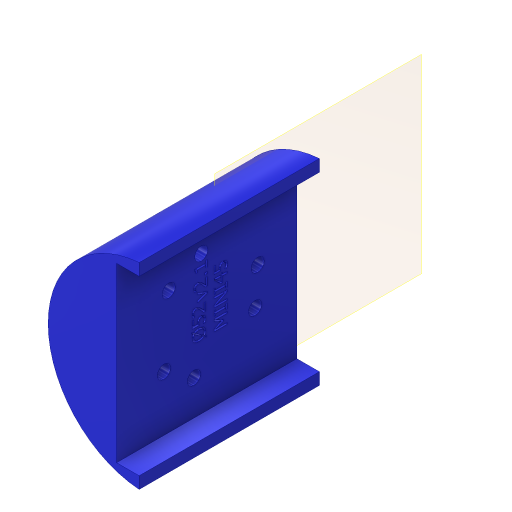
# Autodesk Inventor part: MINI45NewShell52v2-1_A
Saved by Autodesk Inventor 2023 (Build 270158000, 158)
## iProperties
Created: 2016-07-01
Part Number: MINI45NewShell52v2-1_A
Material: ABS Plastic
Document SubType Name: Modeling
Designer: Administrateur
Density: 1.06 g/cm^3
Appearance: Blue - Wall Paint - Glossy
Author: Administrateur
Autodesk Inventor part; units mm, degrees
ref_plane "XZ Plane" through (0, 0, 0) normal (0, 1, 0) x (-1, 0, 0)
sketch "Sketch1" plane through (0, 0, 0) normal (0, 0, 1) x (1, 0, 0)
  arc A0 (0, 26.2509) -> (0, -26.2509) centre (0, 0) ccw
  line L0 (0, 26.2509) -> (0, 23)
  line L1 (0, 23) -> (-8, 23)
  line L2 (-8, 23) -> (-8, 0)
  line L3 (-46.5484, 0) -> (26.4312, 0) construction
  line L4 (0, -26.2509) -> (0, -23)
  line L5 (0, -23) -> (-8, -23)
  line L6 (-8, -23) -> (-8, 0)
  dimension "d2" = 26.2509
  dimension "d3" = 46
  dimension "d4" = 8
  dimension "d27" = 23
  dimension "d28" = 3.2509
  constraints: 14 end point, 2 horizontal, 2 point on circle, 2 symmetric about line, 1 centre point, 1 coincident, 1 perpendicular, 1 vertical
  measures "d2" radius of A0
  measures "d3" distance between parallel lines of L5 L1
  measures "d4" distance of L0.end L1.end
  measures "d27" distance of L1.end L2.end
  measures "d28" distance of L0.start L0.end
extrude "Extrusion1" add sketch "Sketch1" along normal blind 120
sketch "Sketch2" plane through (-8, -23, 0) normal (1, 0, 0) x (0, 0, -1)
  line L0 (-60, 23) -> (-120, 23) construction
  line L1 (-120, 49.2509) -> (-120, -3.2509) construction
  line L2 (0, 49.2509) -> (-120, 49.2509) construction
  line L3 (-60, 49.2509) -> (-60, -3.2509) construction
  line L4 (0, -3.2509) -> (-120, -3.2509) construction
  line L5 (-60, 23) -> (-70.1427, 32.7947) construction
  circle A0 centre (-60, 23) radius 14.1 construction
  line L6 (-60, 23) -> (-61.4739, 37.0228) construction
  line L7 (-60, 23) -> (-63.4111, 9.3188) construction
  line L8 (-60, 23) -> (-71.4071, 14.7122) construction
  line L9 (-60, 23) -> (-46.4462, 26.8865) construction
  line L10 (-60, 23) -> (-47.119, 17.265) construction
  point P0 (0, 23)
  dimension "d32" = 28.2
  dimension "d34" = 40
  dimension "d37" = 360
  dimension "d39" = 84
  constraints: 16 end point, 11 coincident, 4 midpoint, 2 point on circle, 1 centre point, 17 other
  measures "d32" diameter of A0
  measures "d34" angle of L5 L6
  measures "d39" angle of L0 L6
hole "Hole1" at (-8, 14.0228, 61.4739) at (-8, 9.7947, 70.1427) at (-8, -8.2878, 71.4071) at (-8, -13.6812, 63.4111) at (-8, -5.735, 47.119) at (-8, 3.8865, 46.4462) direction (-1, 0, 0) diameter 3.5 end through all
ref_plane "Work Plane1" through (-26.2509, 0, 0) normal (1, 0, 0) x (0, 1, 0)
ref_plane "Work Plane2" through (-10, 0, 0) normal (1, 0, 0) x (0, 1, 0)
ref_plane "Work Plane3" through (-13.3, -23, 0) normal (1, 0, 0) x (0, 0, -1)
sketch "Sketch4" plane through (-13.3, -23, 0) normal (1, 0, 0) x (0, 0, -1)
  line L0 (0, 49.2509) -> (0, -3.2509) projected
  line L1 (0, -3.2509) -> (-120, -3.2509) projected
  line L2 (-120, 49.2509) -> (-120, -3.2509) projected
  line L3 (0, 49.2509) -> (-120, 49.2509) projected
  circle A0 centre (-61.4739, 37.0228) radius 1.75 projected
  circle A1 centre (-70.1427, 32.7947) radius 1.75 projected
  circle A2 centre (-71.4071, 14.7122) radius 1.75 projected
  circle A3 centre (-63.4111, 9.3188) radius 1.75 projected
  circle A4 centre (-47.119, 17.265) radius 1.75 projected
  circle A5 centre (-46.4462, 26.8865) radius 1.75 projected
  point P0 (0, 23)
  point P1 (-47.119, 19.015)
  point P2 (-71.4071, 16.4622)
  point P3 (-61.4739, 38.7728)
  point P4 (-70.1427, 34.5447)
  point P5 (-63.4111, 11.0688)
  point P6 (-46.4462, 28.6365)
  constraints: 6 coincident, 6 vertical alignment, 6 other
hole "Hole3" at (-13.3, 14.0228, 61.4739) at (-13.3, 9.7947, 70.1427) at (-13.3, -8.2878, 71.4071) at (-13.3, -13.6812, 63.4111) at (-13.3, -5.735, 47.119) at (-13.3, 3.8865, 46.4462) direction (-1, 0, 0) diameter 6.5 end through all
sketch "Sketch5" plane through (-8, -23, 0) normal (1, 0, 0) x (0, 0, -1)
  line L0 (-64.0358, 16.8519) -> (-64.0358, 25.5112) construction
  line L1 (-64.0358, 25.5112) -> (-65.8543, 25.5112) construction
  line L2 (-65.8543, 25.5112) -> (-65.8543, 16.8519) construction
  line L3 (-65.8543, 16.8519) -> (-64.0358, 16.8519) construction
  line L4 (-63.4273, 26.0588) -> (-63.4273, 31.0819) construction
  line L5 (-63.4273, 31.0819) -> (-59.8535, 31.0819) construction
  line L6 (-59.8535, 31.0819) -> (-59.8535, 26.0588) construction
  line L7 (-59.8535, 26.0588) -> (-63.4273, 26.0588) construction
  spline S0 degree 2 poles (-62.0703, 20.1023) (-61.2024, 20.1023) (-60.2465, 19.2571) (-60.2465, 18.5537) knots 0 0 0 1 2 2 2
  spline S1 degree 2 poles (-60.2465, 18.5537) (-60.2465, 18.2956) (-60.3827, 17.8503) (-60.5075, 17.6716) knots 0 0 0 1 2 2 2
  line L8 (-60.5075, 17.6716) -> (-60.048, 17.3596)
  line L9 (-60.048, 17.3596) -> (-60.048, 17.0136)
  line L10 (-60.048, 17.0136) -> (-60.7003, 17.4561)
  spline S2 degree 2 poles (-60.7003, 17.4561) (-60.9329, 17.2462) (-61.6193, 17.0079) (-62.0703, 17.0079) knots 0 0 0 1 2 2 2
  spline S3 degree 2 poles (-62.0703, 17.0079) (-62.9353, 17.0079) (-63.894, 17.856) (-63.894, 18.5537) knots 0 0 0 1 2 2 2
  spline S4 degree 2 poles (-63.894, 18.5537) (-63.894, 18.8231) (-63.7635, 19.2429) (-63.6359, 19.4301) knots 0 0 0 1 2 2 2
  line L11 (-63.6359, 19.4301) -> (-64.0358, 19.6996)
  line L12 (-64.0358, 19.6996) -> (-64.0358, 20.0484)
  line L13 (-64.0358, 20.0484) -> (-63.4459, 19.6457)
  spline S5 degree 2 poles (-63.4459, 19.6457) (-63.2133, 19.8612) (-62.5383, 20.1023) (-62.0703, 20.1023) knots 0 0 0 1 2 2 2
  spline S6 degree 2 poles (-62.0703, 19.623) (-62.3936, 19.623) (-62.9013, 19.4925) (-63.0686, 19.3847) knots 0 0 0 1 2 2 2
  line L14 (-63.0686, 19.3847) -> (-60.8648, 17.9099)
  spline S7 degree 2 poles (-60.8648, 17.9099) (-60.7571, 18.0432) (-60.6493, 18.3438) (-60.6493, 18.5565) knots 0 0 0 1 2 2 2
  spline S8 degree 2 poles (-60.6493, 18.5565) (-60.6493, 19.0415) (-61.381, 19.623) (-62.0703, 19.623) knots 0 0 0 1 2 2 2
  spline S9 degree 2 poles (-63.2814, 19.1919) (-63.3863, 19.0699) (-63.4912, 18.7494) (-63.4912, 18.5565) knots 0 0 0 1 2 2 2
  spline S10 degree 2 poles (-63.4912, 18.5565) (-63.4912, 18.0687) (-62.768, 17.4873) (-62.0703, 17.4873) knots 0 0 0 1 2 2 2
  spline S11 degree 2 poles (-62.0703, 17.4873) (-61.7526, 17.4873) (-61.2591, 17.6092) (-61.0832, 17.7198) knots 0 0 0 1 2 2 2
  line L15 (-61.0832, 17.7198) -> (-63.2814, 19.1919)
  spline S12 degree 2 poles (-61.4321, 22.6351) (-61.1797, 22.6351) (-60.7485, 22.4735) (-60.5897, 22.326) knots 0 0 0 1 2 2 2
  spline S13 degree 2 poles (-60.5897, 22.326) (-60.4309, 22.1785) (-60.2465, 21.7389) (-60.2465, 21.4666) knots 0 0 0 1 2 2 2
  spline S14 degree 2 poles (-60.2465, 21.4666) (-60.2465, 21.217) (-60.3571, 20.7291) (-60.4451, 20.5505) knots 0 0 0 1 2 2 2
  line L16 (-60.4451, 20.5505) -> (-60.9414, 20.5505)
  line L17 (-60.9414, 20.5505) -> (-60.9414, 20.5845)
  spline S15 degree 2 poles (-60.9414, 20.5845) (-60.9017, 20.6384) (-60.7996, 20.8398) (-60.7542, 20.9617) knots 0 0 0 1 2 2 2
  spline S16 degree 2 poles (-60.7542, 20.9617) (-60.706, 21.1007) (-60.6521, 21.3304) (-60.6521, 21.4751) knots 0 0 0 1 2 2 2
  spline S17 degree 2 poles (-60.6521, 21.4751) (-60.6521, 21.6169) (-60.7542, 21.8835) (-60.8648, 21.98) knots 0 0 0 1 2 2 2
  spline S18 degree 2 poles (-60.8648, 21.98) (-60.9698, 22.0679) (-61.2477, 22.1586) (-61.4349, 22.1586) knots 0 0 0 1 2 2 2
  spline S19 degree 2 poles (-61.4349, 22.1586) (-61.6221, 22.1586) (-61.8604, 22.0565) (-61.9398, 21.9601) knots 0 0 0 1 2 2 2
  spline S20 degree 2 poles (-61.9398, 21.9601) (-62.0277, 21.8608) (-62.1015, 21.5659) (-62.1015, 21.3872) knots 0 0 0 1 2 2 2
  spline S21 degree 2 poles (-62.1015, 21.3872) (-62.1015, 21.1943) (-62.0419, 20.8114) (-62.0164, 20.6951) knots 0 0 0 1 2 2 2
  line L18 (-62.0164, 20.6951) -> (-63.8203, 20.6951)
  line L19 (-63.8203, 20.6951) -> (-63.8203, 22.6153)
  line L20 (-63.8203, 22.6153) -> (-63.409, 22.6153)
  line L21 (-63.409, 22.6153) -> (-63.409, 21.1461)
  line L22 (-63.409, 21.1461) -> (-62.4759, 21.1461)
  spline S22 degree 2 poles (-62.4759, 21.1461) (-62.4872, 21.2312) (-62.4957, 21.3957) (-62.4957, 21.4637) knots 0 0 0 1 2 2 2
  spline S23 degree 2 poles (-62.4957, 21.4637) (-62.4957, 21.7332) (-62.4078, 22.1048) (-62.2773, 22.2749) knots 0 0 0 1 2 2 2
  spline S24 degree 2 poles (-62.2773, 22.2749) (-62.1468, 22.4479) (-61.7498, 22.6351) (-61.4321, 22.6351) knots 0 0 0 1 2 2 2
  line L23 (-60.3203, 25.2984) -> (-60.3203, 23.14)
  line L24 (-60.3203, 23.14) -> (-60.8166, 23.14)
  spline S25 degree 2 poles (-60.8166, 23.14) (-61.035, 23.3726) (-61.4406, 23.7867) (-61.659, 23.9852) knots 0 0 0 1 2 2 2
  spline S26 degree 2 poles (-61.659, 23.9852) (-62.0986, 24.3851) (-62.6262, 24.6773) (-62.907, 24.6773) knots 0 0 0 1 2 2 2
  spline S27 degree 2 poles (-62.907, 24.6773) (-63.0545, 24.6773) (-63.2757, 24.5865) (-63.3466, 24.5043) knots 0 0 0 1 2 2 2
  spline S28 degree 2 poles (-63.3466, 24.5043) (-63.4175, 24.422) (-63.4884, 24.2065) (-63.4884, 24.076) knots 0 0 0 1 2 2 2
  spline S29 degree 2 poles (-63.4884, 24.076) (-63.4884, 23.9512) (-63.426, 23.6959) (-63.3778, 23.5796) knots 0 0 0 1 2 2 2
  spline S30 degree 2 poles (-63.3778, 23.5796) (-63.3381, 23.4804) (-63.2246, 23.296) (-63.1849, 23.2393) knots 0 0 0 1 2 2 2
  line L25 (-63.1849, 23.2393) -> (-63.1849, 23.2137)
  line L26 (-63.1849, 23.2137) -> (-63.6841, 23.2137)
  spline S31 degree 2 poles (-63.6841, 23.2137) (-63.755, 23.3584) (-63.894, 23.8774) (-63.894, 24.11) knots 0 0 0 1 2 2 2
  spline S32 degree 2 poles (-63.894, 24.11) (-63.894, 24.6007) (-63.375, 25.1538) (-62.9325, 25.1538) knots 0 0 0 1 2 2 2
  spline S33 degree 2 poles (-62.9325, 25.1538) (-62.7254, 25.1538) (-62.3794, 25.0573) (-62.2319, 24.9723) knots 0 0 0 1 2 2 2
  spline S34 degree 2 poles (-62.2319, 24.9723) (-62.0788, 24.8872) (-61.7781, 24.6404) (-61.6335, 24.5043) knots 0 0 0 1 2 2 2
  spline S35 degree 2 poles (-61.6335, 24.5043) (-61.3924, 24.283) (-60.8762, 23.7413) (-60.7259, 23.5796) knots 0 0 0 1 2 2 2
  line L27 (-60.7259, 23.5796) -> (-60.7259, 25.2984)
  line L28 (-60.7259, 25.2984) -> (-60.3203, 25.2984)
  line L29 (-54.5576, 20.2073) -> (-54.5576, 19.7421)
  line L30 (-54.5576, 19.7421) -> (-57.5726, 19.7421)
  line L31 (-57.5726, 19.7421) -> (-55.5219, 18.8288)
  line L32 (-55.5219, 18.8288) -> (-55.5219, 18.5452)
  line L33 (-55.5219, 18.5452) -> (-57.5726, 17.6404)
  line L34 (-57.5726, 17.6404) -> (-54.5576, 17.6404)
  line L35 (-54.5576, 17.6404) -> (-54.5576, 17.2065)
  line L36 (-54.5576, 17.2065) -> (-58.0576, 17.2065)
  line L37 (-58.0576, 17.2065) -> (-58.0576, 17.8418)
  line L38 (-58.0576, 17.8418) -> (-56.1091, 18.7154)
  line L39 (-56.1091, 18.7154) -> (-58.0576, 19.5606)
  line L40 (-58.0576, 19.5606) -> (-58.0576, 20.2073)
  line L41 (-58.0576, 20.2073) -> (-54.5576, 20.2073)
  line L42 (-54.5576, 22.136) -> (-54.5576, 20.7802)
  line L43 (-54.5576, 20.7802) -> (-54.915, 20.7802)
  line L44 (-54.915, 20.7802) -> (-54.915, 21.2255)
  line L45 (-54.915, 21.2255) -> (-57.7002, 21.2255)
  line L46 (-57.7002, 21.2255) -> (-57.7002, 20.7802)
  line L47 (-57.7002, 20.7802) -> (-58.0576, 20.7802)
  line L48 (-58.0576, 20.7802) -> (-58.0576, 22.136)
  line L49 (-58.0576, 22.136) -> (-57.7002, 22.136)
  line L50 (-57.7002, 22.136) -> (-57.7002, 21.6907)
  line L51 (-57.7002, 21.6907) -> (-54.915, 21.6907)
  line L52 (-54.915, 21.6907) -> (-54.915, 22.136)
  line L53 (-54.915, 22.136) -> (-54.5576, 22.136)
  line L54 (-54.5576, 25.2162) -> (-54.5576, 24.6943)
  line L55 (-54.5576, 24.6943) -> (-57.5754, 23.1457)
  line L56 (-57.5754, 23.1457) -> (-54.5576, 23.1457)
  line L57 (-54.5576, 23.1457) -> (-54.5576, 22.7117)
  line L58 (-54.5576, 22.7117) -> (-58.0576, 22.7117)
  line L59 (-58.0576, 22.7117) -> (-58.0576, 23.3726)
  line L60 (-58.0576, 23.3726) -> (-55.2865, 24.7822)
  line L61 (-55.2865, 24.7822) -> (-58.0576, 24.7822)
  line L62 (-58.0576, 24.7822) -> (-58.0576, 25.2162)
  line L63 (-58.0576, 25.2162) -> (-54.5576, 25.2162)
  line L64 (-54.5576, 27.1449) -> (-54.5576, 25.7891)
  line L65 (-54.5576, 25.7891) -> (-54.915, 25.7891)
  line L66 (-54.915, 25.7891) -> (-54.915, 26.2344)
  line L67 (-54.915, 26.2344) -> (-57.7002, 26.2344)
  line L68 (-57.7002, 26.2344) -> (-57.7002, 25.7891)
  line L69 (-57.7002, 25.7891) -> (-58.0576, 25.7891)
  line L70 (-58.0576, 25.7891) -> (-58.0576, 27.1449)
  line L71 (-58.0576, 27.1449) -> (-57.7002, 27.1449)
  line L72 (-57.7002, 27.1449) -> (-57.7002, 26.6996)
  line L73 (-57.7002, 26.6996) -> (-54.915, 26.6996)
  line L74 (-54.915, 26.6996) -> (-54.915, 27.1449)
  line L75 (-54.915, 27.1449) -> (-54.5576, 27.1449)
  line L76 (-55.7602, 29.8734) -> (-55.7602, 29.4565)
  line L77 (-55.7602, 29.4565) -> (-54.5576, 29.4565)
  line L78 (-54.5576, 29.4565) -> (-54.5576, 29.0055)
  line L79 (-54.5576, 29.0055) -> (-55.7602, 29.0055)
  line L80 (-55.7602, 29.0055) -> (-55.7602, 27.4597)
  line L81 (-55.7602, 27.4597) -> (-56.2537, 27.4597)
  line L82 (-56.2537, 27.4597) -> (-58.0576, 29.0253)
  line L83 (-58.0576, 29.0253) -> (-58.0576, 29.4565)
  line L84 (-58.0576, 29.4565) -> (-56.1374, 29.4565)
  line L85 (-56.1374, 29.4565) -> (-56.1374, 29.8734)
  line L86 (-56.1374, 29.8734) -> (-55.7602, 29.8734)
  line L87 (-56.1374, 29.0055) -> (-57.5045, 29.0055)
  line L88 (-57.5045, 29.0055) -> (-56.1374, 27.8284)
  line L89 (-56.1374, 27.8284) -> (-56.1374, 29.0055)
  spline S36 degree 2 poles (-55.6694, 32.3693) (-55.417, 32.3693) (-54.9859, 32.2077) (-54.8271, 32.0602) knots 0 0 0 1 2 2 2
  spline S37 degree 2 poles (-54.8271, 32.0602) (-54.6682, 31.9127) (-54.4839, 31.4731) (-54.4839, 31.2008) knots 0 0 0 1 2 2 2
  spline S38 degree 2 poles (-54.4839, 31.2008) (-54.4839, 30.9512) (-54.5945, 30.4633) (-54.6824, 30.2847) knots 0 0 0 1 2 2 2
  line L90 (-54.6824, 30.2847) -> (-55.1788, 30.2847)
  line L91 (-55.1788, 30.2847) -> (-55.1788, 30.3187)
  spline S39 degree 2 poles (-55.1788, 30.3187) (-55.139, 30.3726) (-55.0369, 30.574) (-54.9916, 30.6959) knots 0 0 0 1 2 2 2
  spline S40 degree 2 poles (-54.9916, 30.6959) (-54.9433, 30.8349) (-54.8895, 31.0646) (-54.8895, 31.2093) knots 0 0 0 1 2 2 2
  spline S41 degree 2 poles (-54.8895, 31.2093) (-54.8895, 31.3511) (-54.9916, 31.6177) (-55.1022, 31.7142) knots 0 0 0 1 2 2 2
  spline S42 degree 2 poles (-55.1022, 31.7142) (-55.2071, 31.8021) (-55.4851, 31.8928) (-55.6723, 31.8928) knots 0 0 0 1 2 2 2
  spline S43 degree 2 poles (-55.6723, 31.8928) (-55.8595, 31.8928) (-56.0977, 31.7907) (-56.1771, 31.6943) knots 0 0 0 1 2 2 2
  spline S44 degree 2 poles (-56.1771, 31.6943) (-56.2651, 31.595) (-56.3388, 31.3001) (-56.3388, 31.1214) knots 0 0 0 1 2 2 2
  spline S45 degree 2 poles (-56.3388, 31.1214) (-56.3388, 30.9285) (-56.2792, 30.5456) (-56.2537, 30.4293) knots 0 0 0 1 2 2 2
  line L92 (-56.2537, 30.4293) -> (-58.0576, 30.4293)
  line L93 (-58.0576, 30.4293) -> (-58.0576, 32.3495)
  line L94 (-58.0576, 32.3495) -> (-57.6463, 32.3495)
  line L95 (-57.6463, 32.3495) -> (-57.6463, 30.8803)
  line L96 (-57.6463, 30.8803) -> (-56.7132, 30.8803)
  spline S46 degree 2 poles (-56.7132, 30.8803) (-56.7245, 30.9654) (-56.733, 31.1299) (-56.733, 31.1979) knots 0 0 0 1 2 2 2
  spline S47 degree 2 poles (-56.733, 31.1979) (-56.733, 31.4674) (-56.6451, 31.839) (-56.5147, 32.0091) knots 0 0 0 1 2 2 2
  spline S48 degree 2 poles (-56.5147, 32.0091) (-56.3842, 32.1821) (-55.9871, 32.3693) (-55.6694, 32.3693) knots 0 0 0 1 2 2 2
  line L97 (-62.48, 28.4413) -> (-59.8535, 27.4514)
  line L98 (-59.8535, 27.4514) -> (-59.8535, 27.0543)
  line L99 (-59.8535, 27.0543) -> (-62.48, 26.073)
  line L100 (-62.48, 26.073) -> (-62.48, 26.5523)
  line L101 (-62.48, 26.5523) -> (-60.4577, 27.2699)
  line L102 (-60.4577, 27.2699) -> (-62.48, 27.9818)
  line L103 (-62.48, 27.9818) -> (-62.48, 28.4413)
  line L104 (-59.8535, 30.8692) -> (-59.8535, 28.7107)
  line L105 (-59.8535, 28.7107) -> (-60.3499, 28.7107)
  spline S49 degree 2 poles (-60.3499, 28.7107) (-60.5683, 28.9433) (-60.9739, 29.3574) (-61.1923, 29.556) knots 0 0 0 1 2 2 2
  spline S50 degree 2 poles (-61.1923, 29.556) (-61.6319, 29.9559) (-62.1595, 30.248) (-62.4403, 30.248) knots 0 0 0 1 2 2 2
  spline S51 degree 2 poles (-62.4403, 30.248) (-62.5877, 30.248) (-62.809, 30.1572) (-62.8799, 30.075) knots 0 0 0 1 2 2 2
  spline S52 degree 2 poles (-62.8799, 30.075) (-62.9508, 29.9927) (-63.0217, 29.7772) (-63.0217, 29.6467) knots 0 0 0 1 2 2 2
  spline S53 degree 2 poles (-63.0217, 29.6467) (-63.0217, 29.5219) (-62.9593, 29.2666) (-62.9111, 29.1504) knots 0 0 0 1 2 2 2
  spline S54 degree 2 poles (-62.9111, 29.1504) (-62.8714, 29.0511) (-62.7579, 28.8667) (-62.7182, 28.81) knots 0 0 0 1 2 2 2
  line L106 (-62.7182, 28.81) -> (-62.7182, 28.7845)
  line L107 (-62.7182, 28.7845) -> (-63.2174, 28.7845)
  spline S55 degree 2 poles (-63.2174, 28.7845) (-63.2883, 28.9291) (-63.4273, 29.4482) (-63.4273, 29.6808) knots 0 0 0 1 2 2 2
  spline S56 degree 2 poles (-63.4273, 29.6808) (-63.4273, 30.1714) (-62.9082, 30.7245) (-62.4658, 30.7245) knots 0 0 0 1 2 2 2
  spline S57 degree 2 poles (-62.4658, 30.7245) (-62.2587, 30.7245) (-61.9127, 30.6281) (-61.7652, 30.543) knots 0 0 0 1 2 2 2
  spline S58 degree 2 poles (-61.7652, 30.543) (-61.6121, 30.4579) (-61.3114, 30.2111) (-61.1668, 30.075) knots 0 0 0 1 2 2 2
  spline S59 degree 2 poles (-61.1668, 30.075) (-60.9257, 29.8538) (-60.4095, 29.312) (-60.2591, 29.1504) knots 0 0 0 1 2 2 2
  line L108 (-60.2591, 29.1504) -> (-60.2591, 30.8692)
  line L109 (-60.2591, 30.8692) -> (-59.8535, 30.8692)
  line L110 (-59.8535, 32.0888) -> (-59.8535, 31.5272)
  line L111 (-59.8535, 31.5272) -> (-60.5229, 31.5272)
  line L112 (-60.5229, 31.5272) -> (-60.5229, 32.0888)
  line L113 (-60.5229, 32.0888) -> (-59.8535, 32.0888)
  line L114 (-59.8535, 34.7776) -> (-59.8535, 33.0701)
  line L115 (-59.8535, 33.0701) -> (-60.2109, 33.0701)
  line L116 (-60.2109, 33.0701) -> (-60.2109, 33.7055)
  line L117 (-60.2109, 33.7055) -> (-62.5565, 33.7055)
  line L118 (-62.5565, 33.7055) -> (-62.5565, 33.0701)
  line L119 (-62.5565, 33.0701) -> (-62.877, 33.0701)
  spline S60 degree 2 poles (-62.877, 33.0701) (-62.877, 33.4303) (-63.0813, 33.7707) (-63.3649, 33.7934) knots 0 0 0 1 2 2 2
  line L120 (-63.3649, 33.7934) -> (-63.3649, 34.1564)
  line L121 (-63.3649, 34.1564) -> (-60.2109, 34.1564)
  line L122 (-60.2109, 34.1564) -> (-60.2109, 34.7776)
  line L123 (-60.2109, 34.7776) -> (-59.8535, 34.7776)
  point P0 (0, 23)
  constraints: 4 other
extrude "Extrusion2" cut sketch "Sketch5" against normal blind 2
sketch "Sketch6" plane through (-8, -23, 0) normal (1, 0, 0) x (0, 0, -1)
  line L0 (-120, 49.2509) -> (-120, -3.2509) projected
  line L1 (0, -3.2509) -> (-120, -3.2509) projected
  line L2 (-120, 49.2509) -> (-84, 49.2509)
  line L3 (-84, 49.2509) -> (-84, -3.2509)
  line L4 (-84, -3.2509) -> (-120, -3.2509)
  line L5 (-120, -3.2509) -> (-120, 49.2509)
  line L6 (0, 49.2509) -> (0, -3.2509) projected
  line L7 (0, 49.2509) -> (-36, 49.2509)
  line L8 (-36, 49.2509) -> (-36, -3.2509)
  line L9 (-36, -3.2509) -> (0, -3.2509)
  line L10 (0, -3.2509) -> (0, 49.2509)
  line L11 (0, 49.2509) -> (-120, 49.2509) construction
  line L12 (-60, 49.2509) -> (-60, -28.4791) construction
  point P0 (0, 23)
  point P1 (-36, -3.2509)
  dimension "d50" = 24
  dimension "d51" = 24
  constraints: 18 end point, 4 parallel, 2 horizontal, 2 perpendicular, 2 point on line, 1 midpoint, 1 vertical
  measures "d50" distance between parallel lines of L8 L12
  measures "d51" distance between parallel lines of L3 L12
extrude "Extrusion3" cut sketch "Sketch6" along normal through all both and the other way through all
sketch "Sketch7" plane through (0, -26.2509, 36) normal (1, 0, 0) x (0, 0, -1)
  line L0 (0, 49.2509) -> (0, 52.5018) projected
  line L1 (0, 52.5018) -> (-48, 52.5018) projected
  line L2 (-48, 52.5018) -> (-48, 49.2509) projected
  line L3 (0, 49.2509) -> (-48, 49.2509) projected
  line L4 (0, 0) -> (0, 3.2509) projected
  line L5 (0, 3.2509) -> (-48, 3.2509) projected
  line L6 (-48, 3.2509) -> (-48, 0) projected
  line L7 (0, 0) -> (-48, 0) projected
  point P0 (36, 26.2509)
extrude "Extrusion4" cut sketch "Sketch7" against normal blind 2
equation "\"d27\" = 0.5 * d3"
equation "\"d28\" = -0.5 * d3 + d2"
equation "\"d51\" = d50"
body "Solid1"
